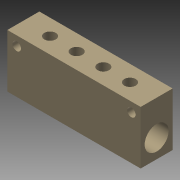
# Autodesk Inventor part: AirVacManifold_v2
Saved by Autodesk Inventor 2015 (Build 190159000, 159)
## iProperties
Created: 2015-03-09
Part Number: AirVacManifold_v2
Material: Generic
Document SubType Name: Modeling
Designer: User
Density: 1 g/cm^3
Appearance: Wheat
Author: User
Autodesk Inventor part; units mm, degrees
ref_plane "YZ Plane" through (0, 0, 0) normal (1, 0, 0) x (0, 1, 0)
sketch "Sketch1" plane through (0, 0, 0) normal (1, 0, 0) x (0, 1, 0)
  line L0 (0, 0) -> (12, 0)
  line L1 (12, 0) -> (12, -20)
  line L2 (12, -20) -> (0, -20)
  line L3 (0, -20) -> (0, 0)
  circle A0 centre (6, -13) radius 4.5
  dimension "d0" = 20
  dimension "d1" = 12
  dimension "d2" = 6
  dimension "d3" = 13
  dimension "d4" = 9
  constraints: 8 end point, 2 parallel, 1 centre point, 1 horizontal, 1 perpendicular
  measures "d0" distance of L0.end L1.end
  measures "d1" distance of L1.end L2.end
  measures "d2" distance from line of L3 A0.centre
  measures "d3" distance from line of L0 A0.centre
  measures "d4" diameter of A0
extrude "Extrusion1" add sketch "Sketch1" against normal blind 50 contours L0 L1 L2 L3 | A0
ref_plane "Work Plane1" through (0, 0, -10) normal (0, 0, 1) x (1, 0, 0)
ref_plane "Work Plane3" through (0, 6, -20) normal (0, -1, 0) x (1, 0, 0)
sketch "Sketch4" plane through (0, 12, 0) normal (0, 1, 0) x (1, 0, 0)
  line L0 (0, 0) -> (0, 20) projected
  line L1 (0, 0) -> (-50, 0) projected
  circle A0 centre (-3.5, 3.5) radius 1.6
  dimension "d93" = 3.2
  dimension "d94" = 3.5
  dimension "d95" = 3.5
  constraints: 1 centre point
  measures "d93" diameter of A0
  measures "d94" distance from line of L1 A0.centre
  measures "d95" distance from line of L0 A0.centre
hole "Hole1" at (0, 6, -13) direction (-1, 0, 0) diameter 9 depth 45
hole "Hole2" at (-3.5, 12, -3.5) direction (0, -1, 0) diameter 3.2 end through all
pattern_linear "Rectangular Pattern7" count 2 spacing 43 along (-1, 0, 0) of "Hole2"
sketch "Sketch2" plane through (0, 0, 0) normal (0, 0, 1) x (1, 0, 0)
  line L0 (0, 0) -> (-50, 0) projected
  line L1 (0, 0) -> (0, 12) projected
  circle A0 centre (-10, 6) radius 2.15
  dimension "d7" = 4.3
  dimension "d8" = 6
  dimension "d9" = 10
  constraints: 1 centre point
  measures "d7" diameter of A0
  measures "d8" distance from line of L0 A0.centre
  measures "d9" distance from line of L1 A0.centre
hole "Hole6" at (-10, 6, 0) direction (0, 0, -1) diameter 4.3 depth 10
pattern_linear "Rectangular Pattern10" count 4 spacing 10 along (-1, 0, 0) of "Hole6"
equation "\"d2\" = 0.5 * d1"
equation "\"d8\" = 0.5 * d1"
body "Solid1"
